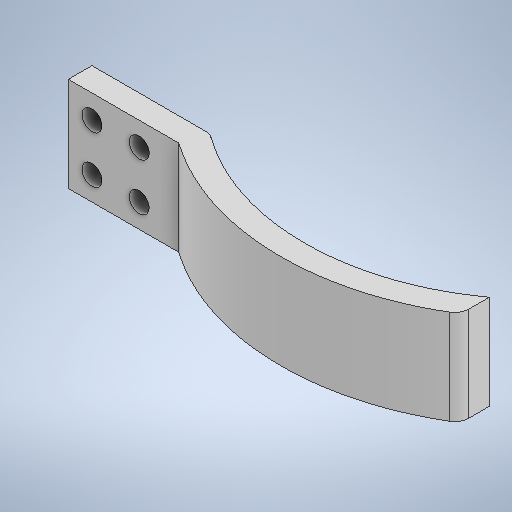
# Autodesk Inventor part: Gripper_Concave_Finger
Saved by Autodesk Inventor 2025.1 (Build 291241000, 241)
## iProperties
Created: 2024-08-03
Part Number: Gripper_Concave_Finger
Material: Generic
Document SubType Name: Modeling
Designer: leonh
Density: 1 g/cm^3
Appearance: Default
Author: leonh
Autodesk Inventor part; units mm, degrees
ref_plane "YZ Plane" through (0, 0, 0) normal (1, 0, 0) x (0, 1, 0)
ref_plane "XZ Plane" through (0, 0, 0) normal (0, 1, 0) x (-1, 0, 0)
ref_plane "XY Plane" through (0, 0, 0) normal (0, 0, 1) x (1, 0, 0)
sketch "Sketch1" plane through (0, 0, 0) normal (0, 1, 0) x (-1, 0, 0)
  line L0 (0, 0) -> (-25, 0)
  spline S0 degree 4 poles (-25, 0) (-32.0397, 5.1858) (-46.8322, 11.6047) (-63.1678, 11.6047) (-77.9603, 5.1858) (-85, 0) knots 0 0 0 0 0 0.5 1 1 1 1 1
  line L1 (-48.6479, 10) -> (-61.3521, 10) construction
  arc A0 (-49.9441, 9.7453) -> (-60.0559, 9.7453) centre (-55, -40.3178) ccw construction
  line L2 (-55, -16.2069) -> (-55, 34.9248) construction
  line L3 (-70, -22.2053) -> (-70, 28.9302) construction
  circle A1 centre (-55, -40) radius 50 construction
  line L4 (-23.3959, 5) -> (0, 5)
  line L5 (-84.476, 6.4124) -> (-84.476, 0)
  line L6 (-84.476, 0) -> (-85, 0)
  line L7 (0, 5) -> (0, 0)
  spline S1 degree 5 poles (-84.476, 6.4124) (-81.1502, 8.5173) (-77.647, 10.3417) (-73.9852, 11.8448) (-65.816, 14.3543) (-57.3038, 15.2371) (-52.6962, 15.2371) (-43.673, 14.3013) (-35.0354, 11.5377) (-30.933, 9.7391) (-27.0473, 7.5377) (-23.3959, 4.9999) knots 0 0 0 0 0 0 0.303739 0.303739 0.303739 0.656836 0.656836 0.656836 1 1 1 1 1 1
  point P0 (-40, 7.697)
  point P1 (-55, 10)
  point P2 (-70, 7.697)
  point P3 (-84.476, 0.3814)
  dimension "d5" = 5
  dimension "d0" = 60
  dimension "d1" = 25
  dimension "d2" = 100
  constraints: 16 end point, 4 point on circle, 3 perpendicular, 2 centre point, 2 horizontal, 2 midpoint, 2 point on line, 2 symmetric about line, 1 horizontal alignment, 1 parallel, 1 vertical, 1 vertical alignment, 9 other
  measures "d0" distance of L6.end L0.end
  measures "d1" distance of L0.start L0.end
  measures "d2" diameter of A1
extrude "Extrusion1" add sketch "Sketch1" along normal blind 20 contours L0 S0 L5 S1 L4 L7
sketch "Sketch2" plane through (25, 0, 0) normal (0, 0, -1) x (-1, 0, 0)
  circle A0 centre (10, 15) radius 2.1
  line L0 (0, 20) -> (25, 20) projected
  line L1 (0, 0) -> (25, 0) projected
  line L2 (25, 0) -> (25, 20) projected
  line L3 (0, 20) -> (25, 20) projected
  line L4 (0, 0) -> (0, 20) projected
  circle A1 centre (20, 15) radius 2.1
  circle A2 centre (10, 5) radius 2.1
  circle A3 centre (20, 5) radius 2.1
  dimension "d8" = 4.2
  dimension "d11" = 10
  dimension "d14" = 10
  dimension "d17" = 10
  dimension "d18" = 5
  constraints: 4 centre point, 1 horizontal, 1 vertical, 6 other
  measures "d8" diameter of A0
  measures "d11" distance of A0.centre A1.centre
  measures "d14" distance of A0.centre A2.centre
  measures "d17" distance from line of L4 A0.centre
  measures "d18" distance from line of L0 A0.centre
extrude "Extrusion2" cut sketch "Sketch2" against normal up to surface (5 mm away) contours A0 | A1 | A2 | A3
fillet "Fillet1" radius 3 1 edges at (84.476, 10, 6.4124)
fillet "Fillet2" radius 2.5 1 edges at (25, 10, 0)
body "Solid1"
